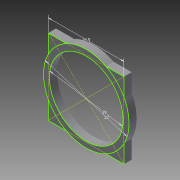
# Autodesk Inventor part: FilterHolder 4x
Saved by Autodesk Inventor 2015 (Build 190159000, 159)
## iProperties
Created: 2015-05-14
Part Number: FilterHolder 4x
Material: Generic
Document SubType Name: Modeling
Designer: Akovo_000
Density: 1 g/cm^3
Appearance: Default
Mass: 1.22106 g
Surface Area: 15.2207 cm^2
Volume: 1.22106 cm^3
Author: Akovo_000
Autodesk Inventor part; units mm, degrees
ref_plane "YZ Plane" through (0, 0, 0) normal (1, 0, 0) x (0, 1, 0)
ref_plane "XZ Plane" through (0, 0, 0) normal (0, 1, 0) x (-1, 0, 0)
ref_plane "XY Plane" through (0, 0, 0) normal (0, 0, 1) x (1, 0, 0)
sketch "Sketch1" plane through (0, 0, 0) normal (0, 1, 0) x (-1, 0, 0)
  line L0 (9.75, -10.7062) -> (5.0929, -10.7062)
  line L1 (-9.75, -10.7062) -> (-9.75, -6.0491)
  line L2 (-9.75, 8.7938) -> (-5.0929, 8.7938)
  line L3 (9.75, 8.7938) -> (9.75, 4.1367)
  line L4 (9.75, -10.7062) -> (-9.75, 8.7938) construction
  line L5 (-9.75, -10.7062) -> (9.75, 8.7938) construction
  circle A0 centre (0, -0.9562) radius 9.5
  circle A1 centre (0, -0.9562) radius 11
  line L6 (5.0929, 8.7938) -> (9.75, 8.7938)
  line L7 (-5.0929, 8.7938) -> (5.0929, 8.7938) construction
  line L8 (-9.75, 4.1367) -> (-9.75, 8.7938)
  line L9 (-9.75, -6.0491) -> (-9.75, 4.1367) construction
  line L10 (-5.0929, -10.7062) -> (-9.75, -10.7062)
  line L11 (5.0929, -10.7062) -> (-5.0929, -10.7062) construction
  line L12 (9.75, -6.0491) -> (9.75, -10.7062)
  line L13 (9.75, 4.1367) -> (9.75, -6.0491) construction
  dimension "d27" = 22
  dimension "d25" = 19.5
  dimension "d26" = 19
  constraints: 28 end point, 18 parallel, 9 perpendicular, 3 horizontal, 2 coincident, 2 midpoint, 1 centre point, 10 other
  measures "d25" distance of L2.start L3.start
  measures "d26" diameter of A0
extrude "Extrusion1" add sketch "Sketch1" along normal blind 2
body "Solid1"
